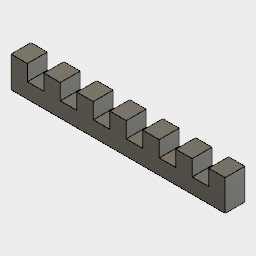
LargeActuator v2 (Autodesk Fusion 360 design; units mm, degrees)
Autodesk Fusion 360 part; units mm, degrees
sketch "Sketch1" plane through (0, 0, 0) normal (0, 1, 0) x (1, 0, 0)
  line L0 (0, 0) -> (88, 0)
  line L1 (88, 0) -> (88, 8.2)
  line L2 (88, 8.2) -> (0, 8.2)
  line L3 (0, 8.2) -> (0, 0)
  dimension "d1" = 88
  dimension "d2" = 8.2
  measures "d1" distance of L0.start L0.end
  measures "d2" distance of L0.start L2.end
extrude "Extrude1" add sketch "Sketch1" along normal blind 12.75
sketch "Sketch2" plane through (0, 12.75, 0) normal (0, 1, 0) x (-1, 0, 0)
  line L0 (0, -8.2) -> (0, 0)
  line L1 (0, 0) -> (-88, 0)
  line L2 (-88, 0) -> (-88, -8.2)
  line L3 (-88, -8.2) -> (0, -8.2)
  line L4 (0, 0) -> (-6.77, 0)
  line L5 (-6.77, 0) -> (-6.77, -8.2)
  line L6 (-6.77, -8.2) -> (0, -8.2)
  line L7 (0, -8.2) -> (0, 0)
  line L8 (-6.77, -8.2) -> (-13.54, -8.2)
  line L9 (-13.54, -8.2) -> (-13.54, 0)
  line L10 (-13.54, 0) -> (-6.77, 0)
  line L11 (-6.77, 0) -> (-6.77, -8.2)
  dimension "d5" = 6.77
  dimension "d6" = 6.77
  measures "d5" distance of L0.end L4.end
  measures "d6" distance of L5.end L8.end
extrude "Extrude2" cut sketch "Sketch2" against normal blind 6.5 contours L1 L3 L5 L8 L9 L10 L11
sketch "Sketch3" plane through (0, 12.75, 0) normal (0, 1, 0) x (-1, 0, 0)
  line L0 (-13.54, -8.2) -> (-13.54, 0)
  line L1 (-13.54, 0) -> (-88, 0)
  line L2 (-88, 0) -> (-88, -8.2)
  line L3 (-88, -8.2) -> (-13.54, -8.2)
  line L4 (-13.54, 0) -> (-20.31, 0)
  line L5 (-20.31, 0) -> (-20.31, -8.2)
  line L6 (-20.31, -8.2) -> (-13.54, -8.2)
  line L7 (-13.54, -8.2) -> (-13.54, 0)
  line L8 (-20.31, -8.2) -> (-27.08, -8.2)
  line L9 (-27.08, -8.2) -> (-27.08, 0)
  line L10 (-27.08, 0) -> (-20.31, 0)
  line L11 (-20.31, 0) -> (-20.31, -8.2)
  dimension "d9" = 6.77
  dimension "d10" = 6.77
  measures "d9" distance of L0.end L4.end
  measures "d10" distance of L5.end L8.end
extrude "Extrude3" cut sketch "Sketch3" against normal blind 6.5 contours L1 L3 L5 L8 L9 L10 L11
sketch "Sketch4" plane through (0, 12.75, 0) normal (0, 1, 0) x (-1, 0, 0)
  line L0 (-27.08, -8.2) -> (-27.08, 0)
  line L1 (-27.08, 0) -> (-88, 0)
  line L2 (-88, 0) -> (-88, -8.2)
  line L3 (-88, -8.2) -> (-27.08, -8.2)
  line L4 (-27.08, 0) -> (-33.85, 0)
  line L5 (-33.85, 0) -> (-33.85, -8.2)
  line L6 (-33.85, -8.2) -> (-27.08, -8.2)
  line L7 (-27.08, -8.2) -> (-27.08, 0)
  line L8 (-33.85, -8.2) -> (-40.62, -8.2)
  line L9 (-40.62, -8.2) -> (-40.62, 0)
  line L10 (-40.62, 0) -> (-33.85, 0)
  line L11 (-33.85, 0) -> (-33.85, -8.2)
  dimension "d13" = 6.77
  dimension "d14" = 6.77
  measures "d13" distance of L0.end L4.end
  measures "d14" distance of L5.end L8.end
extrude "Extrude4" cut sketch "Sketch4" against normal blind 6.5 contours L1 L3 L5 L8 L9 L10 L11
sketch "Sketch5" plane through (0, 12.75, 0) normal (0, 1, 0) x (-1, 0, 0)
  line L0 (-40.62, -8.2) -> (-40.62, 0)
  line L1 (-40.62, 0) -> (-88, 0)
  line L2 (-88, 0) -> (-88, -8.2)
  line L3 (-88, -8.2) -> (-40.62, -8.2)
  line L4 (-40.62, 0) -> (-47.39, 0)
  line L5 (-47.39, 0) -> (-47.39, -8.2)
  line L6 (-47.39, -8.2) -> (-40.62, -8.2)
  line L7 (-40.62, -8.2) -> (-40.62, 0)
  line L8 (-47.39, -8.2) -> (-54.16, -8.2)
  line L9 (-54.16, -8.2) -> (-54.16, 0)
  line L10 (-54.16, 0) -> (-47.39, 0)
  line L11 (-47.39, 0) -> (-47.39, -8.2)
  dimension "d17" = 6.77
  dimension "d18" = 6.77
  measures "d17" distance of L0.end L4.end
  measures "d18" distance of L5.end L8.end
extrude "Extrude5" cut sketch "Sketch5" against normal blind 6.5 contours L1 L3 L5 L8 L9 L10 L11
sketch "Sketch6" plane through (0, 12.75, 0) normal (0, 1, 0) x (-1, 0, 0)
  line L0 (-54.16, -8.2) -> (-54.16, 0)
  line L1 (-54.16, 0) -> (-88, 0)
  line L2 (-88, 0) -> (-88, -8.2)
  line L3 (-88, -8.2) -> (-54.16, -8.2)
  line L4 (-54.16, 0) -> (-60.93, 0)
  line L5 (-60.93, 0) -> (-60.93, -8.2)
  line L6 (-60.93, -8.2) -> (-54.16, -8.2)
  line L7 (-54.16, -8.2) -> (-54.16, 0)
  line L8 (-60.93, 0) -> (-67.7, 0)
  line L9 (-67.7, 0) -> (-67.7, -8.2)
  line L10 (-67.7, -8.2) -> (-60.93, -8.2)
  line L11 (-60.93, -8.2) -> (-60.93, 0)
  dimension "d21" = 6.77
  dimension "d22" = 6.77
  measures "d21" distance of L0.end L4.end
  measures "d22" distance of L4.end L8.end
extrude "Extrude6" cut sketch "Sketch6" against normal blind 6.5 contours L1 L3 L5 L8 L9 L10 L11
sketch "Sketch7" plane through (0, 12.75, 0) normal (0, 1, 0) x (-1, 0, 0)
  line L0 (-67.7, -8.2) -> (-67.7, 0)
  line L1 (-67.7, 0) -> (-88, 0)
  line L2 (-88, 0) -> (-88, -8.2)
  line L3 (-88, -8.2) -> (-67.7, -8.2)
  line L4 (-67.7, 0) -> (-74.47, 0)
  line L5 (-74.47, 0) -> (-74.47, -8.2)
  line L6 (-74.47, -8.2) -> (-67.7, -8.2)
  line L7 (-67.7, -8.2) -> (-67.7, 0)
  line L8 (-74.47, -8.2) -> (-81.24, -8.2)
  line L9 (-81.24, -8.2) -> (-81.24, 0)
  line L10 (-81.24, 0) -> (-74.47, 0)
  line L11 (-74.47, 0) -> (-74.47, -8.2)
  dimension "d25" = 6.77
  dimension "d26" = 6.77
  measures "d25" distance of L0.end L4.end
  measures "d26" distance of L5.end L8.end
extrude "Extrude7" cut sketch "Sketch7" against normal blind 6.5 contours L1 L3 L5 L8 L9 L10 L11
